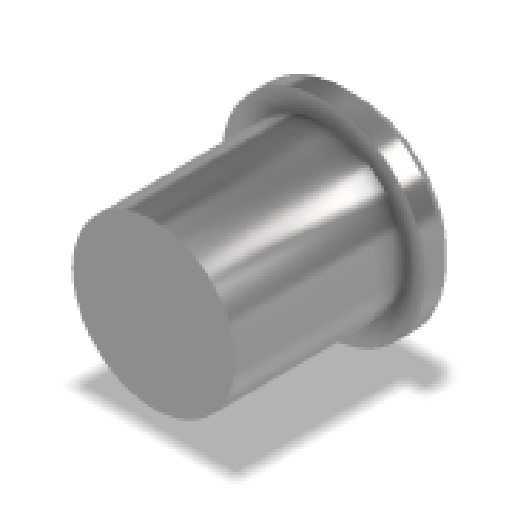
# Autodesk Inventor part: Power Button
Saved by Autodesk Inventor 2023.2 (Build 272271000, 271)
## iProperties
Created: 2023-02-25
Part Number: Power Button
Material: Stainless Steel
Document SubType Name: Modeling
Designer: remop
Density: 8 g/cm^3
Appearance: Semi-Polished
Author: remop
Autodesk Inventor part; units mm, degrees
ref_plane "YZ Plane" through (0, 0, 0) normal (1, 0, 0) x (0, 1, 0)
ref_plane "XZ Plane" through (0, 0, 0) normal (0, 1, 0) x (-1, 0, 0)
ref_plane "XY Plane" through (0, 0, 0) normal (0, 0, 1) x (1, 0, 0)
sketch "Sketch1" plane through (0, 0, 0) normal (1, 0, 0) x (0, 1, 0)
  line L0 (0, 0) -> (8.5858, 0)
  line L1 (8.5858, 0) -> (10, 1.4142)
  line L2 (10, 1.4142) -> (10, 3.4142)
  line L3 (10, 3.4142) -> (8, 3.4142)
  line L4 (8, 3.4142) -> (8, 20)
  line L5 (8, 20) -> (0, 20)
  line L6 (0, 20) -> (0, 0)
  dimension "d1" = 16
  dimension "d2" = 2
  dimension "d3" = 2
  dimension "d4" = 45
  dimension "d5" = 20
  constraints: 14 end point, 5 perpendicular, 1 equal length, 1 horizontal
  measures "d1" diameter of L4 L6
  measures "d2" distance of L2.end L3.end
  measures "d3" distance of L1.end L2.end
  measures "d4" angle of L2 L1
  measures "d5" distance of L5.end L0.start
revolve "Revolution1" add sketch "Sketch1" angle 360 about axis through (0, 0, 20) along (0, 0, -1)
sketch "Sketch2" plane through (0, 0, 0) normal (0, 0, -1) x (-1, 0, 0)
  circle A0 centre (0, 0) radius 8.5858 projected
  circle A1 centre (0, 0) radius 8.0858
  circle A2 centre (0, 0) radius 7.0858
  dimension "d7" = 0.5
  dimension "d8" = 1
  constraints: 2 centre point, 2 coincident
  measures "d7" radial gap between concentric circles of A0 A1
  measures "d8" radial gap between concentric circles of A1 A2
extrude "Extrusion1" cut sketch "Sketch2" against normal blind 0.1 contours A1
body "Solid1"
